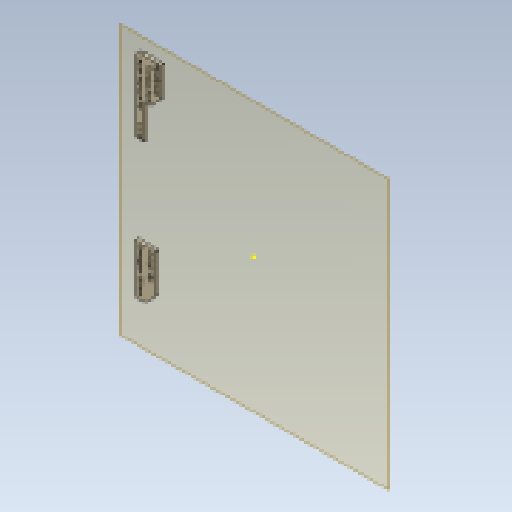
# Autodesk Inventor part: V4-tag
Saved by Autodesk Inventor 2023 (Build 270158030, 158C)
## iProperties
Created: 2024-12-31
Part Number: V4-tag
Material: Generic
Document SubType Name: Modeling
Designer: Imogen Heard
Density: 1 g/cm^3
Appearance: Default
Author: Imogen Heard
Autodesk Inventor part; units mm, degrees
(part 1 of 2)
ref_plane "YZ Plane" through (0, 0, 0) normal (1, 0, 0) x (0, 1, 0)
ref_plane "XZ Plane" through (0, 0, 0) normal (0, 1, 0) x (-1, 0, 0)
ref_plane "XY Plane" through (0, 0, 0) normal (0, 0, 1) x (1, 0, 0)
ref_plane "Work Plane1" through (0, 0, 0) normal (0, 0, 1) x (1, 0, 0)
sketch "Sketch1" plane through (0, 0, 0) normal (0, 0, 1) x (1, 0, 0)
  arc A0 (-110, 115) -> (-115, 110) centre (-110, 110) ccw projected
  line L0 (-115, 110) -> (-115, -110) projected
  arc A1 (-115, -110) -> (-110, -115) centre (-110, -110) ccw projected
  line L1 (-110, -115) -> (110, -115) projected
  arc A2 (110, -115) -> (115, -110) centre (110, -110) ccw projected
  line L2 (115, -110) -> (115, 110) projected
  arc A3 (115, 110) -> (110, 115) centre (110, 110) ccw projected
  line L3 (110, 115) -> (-110, 115) projected
  line L4 (-112, -107) -> (-112, 107) projected
  arc A4 (-107, 112) -> (-112, 107) centre (-107, 107) ccw projected
  line L5 (-107, 112) -> (107, 112) projected
  arc A5 (112, 107) -> (107, 112) centre (107, 107) ccw projected
  line L6 (112, 107) -> (112, -107) projected
  arc A6 (107, -112) -> (112, -107) centre (107, -107) ccw projected
  line L7 (107, -112) -> (-107, -112) projected
  arc A7 (-112, -107) -> (-107, -112) centre (-107, -107) ccw projected
  line L8 (-112, 106.9171) -> (-103.6459, 106.9171)
  line L9 (-103.6459, 106.9171) -> (-103.6459, 42)
  line L10 (-103.6459, 42) -> (-112, 42)
  line L11 (-112, 42) -> (-112, 106.9171)
  line L12 (-87.4562, 112) -> (-103.6459, 112)
  line L13 (-103.6459, 112) -> (-103.6459, 74.4586)
  line L14 (-103.6459, 74.4586) -> (-87.4562, 74.4586)
  line L15 (-87.4562, 74.4586) -> (-87.4562, 112)
  line L16 (-112, -88.3406) -> (-103.6459, -88.3406)
  line L17 (-103.6459, -88.3406) -> (-103.6459, -20.4572)
  line L18 (-103.6459, -20.4572) -> (-112, -20.4572)
  line L19 (-112, -20.4572) -> (-112, -88.3406)
  line L20 (-103.6459, -88.3406) -> (-92.5687, -88.3406)
  line L21 (-92.5687, -88.3406) -> (-92.5687, -42.0436)
  line L22 (-92.5687, -42.0436) -> (-103.6459, -42.0436)
  line L23 (-103.6459, -42.0436) -> (-103.6459, -88.3406)
  line L24 (-103.6459, -42.0436) -> (-112, -42.0436)
  point P0 (0, 0)
  point P1 (-112, 42)
  dimension "d0" = 19.4313
  dimension "d1" = 23.6594
  dimension "d2" = 67.8835
  dimension "d3" = 8.3541
  dimension "d4" = 46.2971
  dimension "d5" = 37.5414
  dimension "d6" = 24.5438
  dimension "d7" = 70
  constraints: 34 end point, 8 parallel, 5 perpendicular, 4 horizontal, 3 point on line, 1 midpoint, 1 vertical alignment
  measures "d0" distance between parallel lines of L4 L21
  measures "d1" distance between parallel lines of L7 L20
  measures "d2" distance between parallel lines of L16 L18
  measures "d3" distance between parallel lines of L4 L17
  measures "d4" distance between parallel lines of L20 L22
  measures "d5" distance between parallel lines of L14 L5
  measures "d6" distance between parallel lines of L4 L15
  measures "d7" distance between parallel lines of L5 L10
ref_plane "Work Plane2" through (-115, -115, -3) normal (0, 0, -1) x (0, 1, 0)
extrude "Extrusion1" add sketch "Sketch1" against normal up to surface (3 mm away) contours L4 L24 L17 L16 | L17 L22 L21 L20 | L4 L8 L9 L10 | L4 A4 L5 L13 L8 | L13 L5 L15 L14 L9
sketch "Sketch2" plane through (0, 0, 0) normal (0, 0, 1) x (1, 0, 0)
  line L0 (-96.6325, 106.512) -> (-96.6325, 80.11) construction
  line L1 (-96.6325, 80.11) -> (-101.6576, 80.11) construction
  line L2 (-101.6576, 80.11) -> (-101.6576, 106.512) construction
  line L3 (-101.6576, 106.512) -> (-96.6325, 106.512) construction
  line L4 (-104.2392, -43.9733) -> (-104.2392, -87.8328) construction
  line L5 (-104.2392, -87.8328) -> (-109.5674, -87.8328) construction
  line L6 (-109.5674, -87.8328) -> (-109.5674, -43.9733) construction
  line L7 (-109.5674, -43.9733) -> (-104.2392, -43.9733) construction
  line L8 (-105.1294, 107.7909) -> (-105.1294, 58.4425) construction
  line L9 (-105.1294, 58.4425) -> (-111.7495, 58.4425) construction
  line L10 (-111.7495, 58.4425) -> (-111.7495, 107.7909) construction
  line L11 (-111.7495, 107.7909) -> (-105.1294, 107.7909) construction
  line L12 (-111.4099, 55.2755) -> (-105.5419, 55.2755) construction
  line L13 (-105.5419, 55.2755) -> (-105.5419, 39.3946) construction
  line L14 (-105.5419, 39.3946) -> (-111.4099, 39.3946) construction
  line L15 (-111.4099, 39.3946) -> (-111.4099, 55.2755) construction
  line L16 (-88.9713, 111.3431) -> (-88.9713, 84.8277) construction
  line L17 (-88.9713, 84.8277) -> (-94.2996, 84.8277) construction
  line L18 (-94.2996, 84.8277) -> (-94.2996, 111.3431) construction
  line L19 (-94.2996, 111.3431) -> (-88.9713, 111.3431) construction
  line L20 (-101.2537, -44.3446) -> (-95.3445, -44.3446) construction
  line L21 (-95.3445, -44.3446) -> (-95.3445, -74.0743) construction
  line L22 (-95.3445, -74.0743) -> (-101.2537, -74.0743) construction
  line L23 (-101.2537, -74.0743) -> (-101.2537, -44.3446) construction
  line L24 (-94.1942, 106.5497) -> (-94.1942, 107.2142)
  line L25 (-94.1942, 107.2142) -> (-89.8871, 107.2142)
  line L26 (-89.8871, 107.2142) -> (-92.8166, 108.5189)
  line L27 (-92.8166, 108.5189) -> (-92.8166, 108.9241)
  line L28 (-92.8166, 108.9241) -> (-89.8871, 110.2166)
  line L29 (-89.8871, 110.2166) -> (-94.1942, 110.2166)
  line L30 (-94.1942, 110.2166) -> (-94.1942, 110.8366)
  line L31 (-94.1942, 110.8366) -> (-89.1942, 110.8366)
  line L32 (-89.1942, 110.8366) -> (-89.1942, 109.929)
  line L33 (-89.1942, 109.929) -> (-91.9778, 108.681)
  line L34 (-91.9778, 108.681) -> (-89.1942, 107.4735)
  line L35 (-89.1942, 107.4735) -> (-89.1942, 106.5497)
  line L36 (-89.1942, 106.5497) -> (-94.1942, 106.5497)
  spline S0 degree 2 poles (-94.2793, 103.9565) (-94.2793, 104.856) (-93.2704, 105.8447) (-92.3384, 105.8447) knots 0 0 0 1 2 2 2
  spline S1 degree 2 poles (-92.3384, 105.8447) (-91.4227, 105.8447) (-90.3368, 104.8844) (-90.3368, 104.1105) knots 0 0 0 1 2 2 2
  spline S2 degree 2 poles (-90.3368, 104.1105) (-90.3368, 103.762) (-90.5394, 103.2231) (-90.7542, 103.0246) knots 0 0 0 1 2 2 2
  spline S3 degree 2 poles (-90.7542, 103.0246) (-90.9689, 102.822) (-91.5889, 102.6072) (-92.0386, 102.6072) knots 0 0 0 1 2 2 2
  line L37 (-92.0386, 102.6072) -> (-92.383, 102.6072)
  line L38 (-92.383, 102.6072) -> (-92.383, 105.2045)
  spline S4 degree 2 poles (-92.383, 105.2045) (-93.0354, 105.2045) (-93.7282, 104.5481) (-93.7282, 103.9646) knots 0 0 0 1 2 2 2
  spline S5 degree 2 poles (-93.7282, 103.9646) (-93.7282, 103.758) (-93.635, 103.3568) (-93.5621, 103.1948) knots 0 0 0 1 2 2 2
  spline S6 degree 2 poles (-93.5621, 103.1948) (-93.4811, 103.0246) (-93.3393, 102.7896) (-93.2744, 102.7126) knots 0 0 0 1 2 2 2
  line L39 (-93.2744, 102.7126) -> (-93.2744, 102.6761)
  line L40 (-93.2744, 102.6761) -> (-93.9632, 102.6761)
  spline S7 degree 2 poles (-93.9632, 102.6761) (-94.0078, 102.7855) (-94.1375, 103.1178) (-94.1739, 103.2474) knots 0 0 0 1 2 2 2
  spline S8 degree 2 poles (-94.1739, 103.2474) (-94.2266, 103.4298) (-94.2793, 103.7296) (-94.2793, 103.9565) knots 0 0 0 1 2 2 2
  spline S9 degree 2 poles (-91.9008, 103.2231) (-91.6456, 103.2312) (-91.2728, 103.3366) (-91.1472, 103.4379) knots 0 0 0 1 2 2 2
  spline S10 degree 2 poles (-91.1472, 103.4379) (-91.0054, 103.5473) (-90.8555, 103.8917) (-90.8555, 104.147) knots 0 0 0 1 2 2 2
  spline S11 degree 2 poles (-90.8555, 104.147) (-90.8555, 104.3982) (-91.0054, 104.7507) (-91.1513, 104.8965) knots 0 0 0 1 2 2 2
  spline S12 degree 2 poles (-91.1513, 104.8965) (-91.3012, 105.0384) (-91.6618, 105.1842) (-91.9008, 105.2045) knots 0 0 0 1 2 2 2
  line L41 (-91.9008, 105.2045) -> (-91.9008, 103.2231)
  line L42 (-94.1942, 99.0821) -> (-94.1942, 99.7142)
  line L43 (-94.1942, 99.7142) -> (-93.8133, 99.7142)
  spline S13 degree 2 poles (-93.8133, 99.7142) (-93.9349, 99.8601) (-94.097, 100.0748) (-94.1658, 100.2207) knots 0 0 0 1 2 2 2
  spline S14 degree 2 poles (-94.1658, 100.2207) (-94.2307, 100.3544) (-94.2996, 100.6421) (-94.2996, 100.8325) knots 0 0 0 1 2 2 2
  spline S15 degree 2 poles (-94.2996, 100.8325) (-94.2996, 101.1405) (-94.0443, 101.6591) (-93.7971, 101.8414) knots 0 0 0 1 2 2 2
  spline S16 degree 2 poles (-93.7971, 101.8414) (-93.55, 102.0238) (-92.8206, 102.2264) (-92.3466, 102.2264) knots 0 0 0 1 2 2 2
  spline S17 degree 2 poles (-92.3466, 102.2264) (-91.8522, 102.2264) (-91.131, 101.9711) (-90.8595, 101.7483) knots 0 0 0 1 2 2 2
  spline S18 degree 2 poles (-90.8595, 101.7483) (-90.6164, 101.5416) (-90.3368, 100.9622) (-90.3368, 100.6421) knots 0 0 0 1 2 2 2
  spline S19 degree 2 poles (-90.3368, 100.6421) (-90.3368, 100.3625) (-90.4624, 99.9452) (-90.5921, 99.7142) knots 0 0 0 1 2 2 2
  line L44 (-90.5921, 99.7142) -> (-88.9713, 99.7142)
  line L45 (-88.9713, 99.7142) -> (-88.9713, 99.0821)
  line L46 (-88.9713, 99.0821) -> (-94.1942, 99.0821)
  line L47 (-93.2825, 99.7142) -> (-91.1148, 99.7142)
  spline S20 degree 2 poles (-91.1148, 99.7142) (-91.0013, 99.9492) (-90.9162, 100.322) (-90.9162, 100.5367) knots 0 0 0 1 2 2 2
  spline S21 degree 2 poles (-90.9162, 100.5367) (-90.9162, 101.023) (-91.6456, 101.574) (-92.3344, 101.574) knots 0 0 0 1 2 2 2
  spline S22 degree 2 poles (-92.3344, 101.574) (-92.9989, 101.574) (-93.6999, 101.1526) (-93.6999, 100.6867) knots 0 0 0 1 2 2 2
  spline S23 degree 2 poles (-93.6999, 100.6867) (-93.6999, 100.4395) (-93.473, 99.9371) (-93.2825, 99.7142) knots 0 0 0 1 2 2 2
  line L48 (-94.1942, 97.5222) -> (-94.1942, 98.1542)
  line L49 (-94.1942, 98.1542) -> (-90.4422, 98.1542)
  line L50 (-90.4422, 98.1542) -> (-90.4422, 97.5222)
  line L51 (-90.4422, 97.5222) -> (-94.1942, 97.5222)
  line L52 (-89.8182, 97.4776) -> (-89.8182, 98.1948)
  line L53 (-89.8182, 98.1948) -> (-89.1618, 98.1948)
  line L54 (-89.1618, 98.1948) -> (-89.1618, 97.4776)
  line L55 (-89.1618, 97.4776) -> (-89.8182, 97.4776)
  spline S24 degree 2 poles (-94.2793, 94.9654) (-94.2793, 95.8649) (-93.2704, 96.8536) (-92.3384, 96.8536) knots 0 0 0 1 2 2 2
  spline S25 degree 2 poles (-92.3384, 96.8536) (-91.4227, 96.8536) (-90.3368, 95.8933) (-90.3368, 95.1194) knots 0 0 0 1 2 2 2
  spline S26 degree 2 poles (-90.3368, 95.1194) (-90.3368, 94.7709) (-90.5394, 94.232) (-90.7542, 94.0335) knots 0 0 0 1 2 2 2
  spline S27 degree 2 poles (-90.7542, 94.0335) (-90.9689, 93.8309) (-91.5889, 93.6162) (-92.0386, 93.6162) knots 0 0 0 1 2 2 2
  line L56 (-92.0386, 93.6162) -> (-92.383, 93.6162)
  line L57 (-92.383, 93.6162) -> (-92.383, 96.2134)
  spline S28 degree 2 poles (-92.383, 96.2134) (-93.0354, 96.2134) (-93.7282, 95.557) (-93.7282, 94.9735) knots 0 0 0 1 2 2 2
  spline S29 degree 2 poles (-93.7282, 94.9735) (-93.7282, 94.7669) (-93.635, 94.3658) (-93.5621, 94.2037) knots 0 0 0 1 2 2 2
  spline S30 degree 2 poles (-93.5621, 94.2037) (-93.4811, 94.0335) (-93.3393, 93.7985) (-93.2744, 93.7215) knots 0 0 0 1 2 2 2
  line L58 (-93.2744, 93.7215) -> (-93.2744, 93.685)
  line L59 (-93.2744, 93.685) -> (-93.9632, 93.685)
  spline S31 degree 2 poles (-93.9632, 93.685) (-94.0078, 93.7944) (-94.1375, 94.1267) (-94.1739, 94.2564) knots 0 0 0 1 2 2 2
  spline S32 degree 2 poles (-94.1739, 94.2564) (-94.2266, 94.4387) (-94.2793, 94.7385) (-94.2793, 94.9654) knots 0 0 0 1 2 2 2
  spline S33 degree 2 poles (-91.9008, 94.232) (-91.6456, 94.2401) (-91.2728, 94.3455) (-91.1472, 94.4468) knots 0 0 0 1 2 2 2
  spline S34 degree 2 poles (-91.1472, 94.4468) (-91.0054, 94.5562) (-90.8555, 94.9006) (-90.8555, 95.1559) knots 0 0 0 1 2 2 2
  spline S35 degree 2 poles (-90.8555, 95.1559) (-90.8555, 95.4071) (-91.0054, 95.7596) (-91.1513, 95.9055) knots 0 0 0 1 2 2 2
  spline S36 degree 2 poles (-91.1513, 95.9055) (-91.3012, 96.0473) (-91.6618, 96.1931) (-91.9008, 96.2134) knots 0 0 0 1 2 2 2
  line L60 (-91.9008, 96.2134) -> (-91.9008, 94.232)
  line L61 (-90.4422, 90.0303) -> (-94.1942, 91.4444)
  line L62 (-94.1942, 91.4444) -> (-94.1942, 92.0116)
  line L63 (-94.1942, 92.0116) -> (-90.4422, 93.4136)
  line L64 (-90.4422, 93.4136) -> (-90.4422, 92.7288)
  line L65 (-90.4422, 92.7288) -> (-93.3312, 91.7037)
  line L66 (-93.3312, 91.7037) -> (-90.4422, 90.6867)
  line L67 (-90.4422, 90.6867) -> (-90.4422, 90.0303)
  spline S37 degree 2 poles (-93.7971, 87.4614) (-93.8538, 87.5384) (-94.0564, 87.7977) (-94.1172, 87.9192) knots 0 0 0 1 2 2 2
  spline S38 degree 2 poles (-94.1172, 87.9192) (-94.2064, 88.0854) (-94.2996, 88.3974) (-94.2996, 88.681) knots 0 0 0 1 2 2 2
  spline S39 degree 2 poles (-94.2996, 88.681) (-94.2996, 88.9119) (-94.1253, 89.3293) (-93.9673, 89.4873) knots 0 0 0 1 2 2 2
  spline S40 degree 2 poles (-93.9673, 89.4873) (-93.8133, 89.6372) (-93.3595, 89.8196) (-93.1083, 89.8196) knots 0 0 0 1 2 2 2
  spline S41 degree 2 poles (-93.1083, 89.8196) (-92.7193, 89.8196) (-92.1683, 89.4914) (-92.0102, 89.1348) knots 0 0 0 1 2 2 2
  spline S42 degree 2 poles (-92.0102, 89.1348) (-91.8644, 88.8188) (-91.755, 87.9598) (-91.7266, 87.4614) knots 0 0 0 1 2 2 2
  line L68 (-91.7266, 87.4614) -> (-91.6051, 87.4614)
  spline S43 degree 2 poles (-91.6051, 87.4614) (-91.3863, 87.4614) (-91.1148, 87.5951) (-91.0378, 87.7166) knots 0 0 0 1 2 2 2
  spline S44 degree 2 poles (-91.0378, 87.7166) (-90.9608, 87.8382) (-90.9122, 88.1867) (-90.9122, 88.373) knots 0 0 0 1 2 2 2
  spline S45 degree 2 poles (-90.9122, 88.373) (-90.9122, 88.5918) (-91.0419, 89.1834) (-91.1675, 89.4792) knots 0 0 0 1 2 2 2
  line L69 (-91.1675, 89.4792) -> (-91.1675, 89.5157)
  line L70 (-91.1675, 89.5157) -> (-90.5232, 89.5157)
  spline S46 degree 2 poles (-90.5232, 89.5157) (-90.4746, 89.3414) (-90.353, 88.6891) (-90.353, 88.369) knots 0 0 0 1 2 2 2
  spline S47 degree 2 poles (-90.353, 88.369) (-90.353, 87.98) (-90.4746, 87.4492) (-90.6326, 87.2385) knots 0 0 0 1 2 2 2
  spline S48 degree 2 poles (-90.6326, 87.2385) (-90.7866, 87.0319) (-91.2769, 86.8293) (-91.6294, 86.8293) knots 0 0 0 1 2 2 2
  line L71 (-91.6294, 86.8293) -> (-94.1942, 86.8293)
  line L72 (-94.1942, 86.8293) -> (-94.1942, 87.4614)
  line L73 (-94.1942, 87.4614) -> (-93.7971, 87.4614)
  line L74 (-93.2704, 87.4614) -> (-92.229, 87.4614)
  spline S49 degree 2 poles (-92.229, 87.4614) (-92.2493, 87.6883) (-92.3182, 88.373) (-92.383, 88.5878) knots 0 0 0 1 2 2 2
  spline S50 degree 2 poles (-92.383, 88.5878) (-92.46, 88.839) (-92.7801, 89.1672) (-93.0637, 89.1672) knots 0 0 0 1 2 2 2
  spline S51 degree 2 poles (-93.0637, 89.1672) (-93.3879, 89.1672) (-93.7161, 88.8025) (-93.7161, 88.4541) knots 0 0 0 1 2 2 2
  spline S52 degree 2 poles (-93.7161, 88.4541) (-93.7161, 88.1583) (-93.4608, 87.6721) (-93.2704, 87.4614) knots 0 0 0 1 2 2 2
  line L75 (-94.1942, 85.2977) -> (-94.1942, 85.9298)
  line L76 (-94.1942, 85.9298) -> (-88.9713, 85.9298)
  line L77 (-88.9713, 85.9298) -> (-88.9713, 85.2977)
  line L78 (-88.9713, 85.2977) -> (-94.1942, 85.2977)
  line L79 (-101.8554, 104.8386) -> (-97.447, 104.8386)
  line L80 (-97.447, 104.8386) -> (-97.447, 106.5161)
  line L81 (-97.447, 106.5161) -> (-96.8554, 106.5161)
  line L82 (-96.8554, 106.5161) -> (-96.8554, 102.4966)
  line L83 (-96.8554, 102.4966) -> (-97.447, 102.4966)
  line L84 (-97.447, 102.4966) -> (-97.447, 104.1741)
  line L85 (-97.447, 104.1741) -> (-101.8554, 104.1741)
  line L86 (-101.8554, 104.1741) -> (-101.8554, 104.8386)
  line L87 (-98.78, 100.0493) -> (-98.78, 100.0817)
  spline S53 degree 2 poles (-98.78, 100.0817) (-98.7598, 100.1547) (-98.7517, 100.3127) (-98.7517, 100.4221) knots 0 0 0 1 2 2 2
  spline S54 degree 2 poles (-98.7517, 100.4221) (-98.7517, 100.6773) (-98.9745, 101.1798) (-99.1933, 101.4067) knots 0 0 0 1 2 2 2
  line L88 (-99.1933, 101.4067) -> (-101.8554, 101.4067)
  line L89 (-101.8554, 101.4067) -> (-101.8554, 102.0388)
  line L90 (-101.8554, 102.0388) -> (-98.1034, 102.0388)
  line L91 (-98.1034, 102.0388) -> (-98.1034, 101.4067)
  line L92 (-98.1034, 101.4067) -> (-98.6625, 101.4067)
  spline S55 degree 2 poles (-98.6625, 101.4067) (-98.3546, 101.0623) (-98.1034, 100.5477) (-98.1034, 100.3046) knots 0 0 0 1 2 2 2
  spline S56 degree 2 poles (-98.1034, 100.3046) (-98.1034, 100.2073) (-98.1115, 100.1101) (-98.1236, 100.0493) knots 0 0 0 1 2 2 2
  line L93 (-98.1236, 100.0493) -> (-98.78, 100.0493)
  spline S57 degree 2 poles (-101.9405, 97.9302) (-101.9405, 98.8297) (-100.9316, 99.8184) (-99.9996, 99.8184) knots 0 0 0 1 2 2 2
  spline S58 degree 2 poles (-99.9996, 99.8184) (-99.0839, 99.8184) (-97.998, 98.8581) (-97.998, 98.0842) knots 0 0 0 1 2 2 2
  spline S59 degree 2 poles (-97.998, 98.0842) (-97.998, 97.7357) (-98.2006, 97.1968) (-98.4154, 96.9983) knots 0 0 0 1 2 2 2
  spline S60 degree 2 poles (-98.4154, 96.9983) (-98.6301, 96.7957) (-99.25, 96.5809) (-99.6998, 96.5809) knots 0 0 0 1 2 2 2
  line L94 (-99.6998, 96.5809) -> (-100.0442, 96.5809)
  line L95 (-100.0442, 96.5809) -> (-100.0442, 99.1782)
  spline S61 degree 2 poles (-100.0442, 99.1782) (-100.6966, 99.1782) (-101.3894, 98.5218) (-101.3894, 97.9383) knots 0 0 0 1 2 2 2
  spline S62 degree 2 poles (-101.3894, 97.9383) (-101.3894, 97.7316) (-101.2962, 97.3305) (-101.2233, 97.1684) knots 0 0 0 1 2 2 2
  spline S63 degree 2 poles (-101.2233, 97.1684) (-101.1423, 96.9983) (-101.0005, 96.7632) (-100.9356, 96.6863) knots 0 0 0 1 2 2 2
  line L96 (-100.9356, 96.6863) -> (-100.9356, 96.6498)
  line L97 (-100.9356, 96.6498) -> (-101.6244, 96.6498)
  spline S64 degree 2 poles (-101.6244, 96.6498) (-101.669, 96.7592) (-101.7987, 97.0914) (-101.8351, 97.2211) knots 0 0 0 1 2 2 2
  spline S65 degree 2 poles (-101.8351, 97.2211) (-101.8878, 97.4034) (-101.9405, 97.7033) (-101.9405, 97.9302) knots 0 0 0 1 2 2 2
  spline S66 degree 2 poles (-99.562, 97.1968) (-99.3068, 97.2049) (-98.934, 97.3102) (-98.8084, 97.4115) knots 0 0 0 1 2 2 2
  spline S67 degree 2 poles (-98.8084, 97.4115) (-98.6666, 97.5209) (-98.5167, 97.8654) (-98.5167, 98.1206) knots 0 0 0 1 2 2 2
  spline S68 degree 2 poles (-98.5167, 98.1206) (-98.5167, 98.3718) (-98.6666, 98.7244) (-98.8124, 98.8702) knots 0 0 0 1 2 2 2
  spline S69 degree 2 poles (-98.8124, 98.8702) (-98.9624, 99.012) (-99.323, 99.1579) (-99.562, 99.1782) knots 0 0 0 1 2 2 2
  line L98 (-99.562, 99.1782) -> (-99.562, 97.1968)
  spline S70 degree 2 poles (-99.9186, 92.7965) (-100.8384, 92.7965) (-101.9607, 93.6879) (-101.9607, 94.3605) knots 0 0 0 1 2 2 2
  spline S71 degree 2 poles (-101.9607, 94.3605) (-101.9607, 94.6644) (-101.8108, 95.0979) (-101.6812, 95.3086) knots 0 0 0 1 2 2 2
  line L99 (-101.6812, 95.3086) -> (-101.8554, 95.3491)
  line L100 (-101.8554, 95.3491) -> (-101.8554, 95.9407)
  line L101 (-101.8554, 95.9407) -> (-96.6325, 95.9407)
  line L102 (-96.6325, 95.9407) -> (-96.6325, 95.3086)
  line L103 (-96.6325, 95.3086) -> (-98.4964, 95.3086)
  spline S72 degree 2 poles (-98.4964, 95.3086) (-98.2816, 95.0696) (-97.998, 94.5145) (-97.998, 94.162) knots 0 0 0 1 2 2 2
  spline S73 degree 2 poles (-97.998, 94.162) (-97.998, 93.5258) (-99.015, 92.7965) (-99.9186, 92.7965) knots 0 0 0 1 2 2 2
  spline S74 degree 2 poles (-99.9672, 93.4488) (-99.2946, 93.4488) (-98.5977, 93.8581) (-98.5977, 94.3119) knots 0 0 0 1 2 2 2
  spline S75 degree 2 poles (-98.5977, 94.3119) (-98.5977, 94.5671) (-98.8408, 95.0939) (-99.0272, 95.3086) knots 0 0 0 1 2 2 2
  line L104 (-99.0272, 95.3086) -> (-101.1787, 95.3086)
  spline S76 degree 2 poles (-101.1787, 95.3086) (-101.2962, 95.0696) (-101.3935, 94.7008) (-101.3935, 94.482) knots 0 0 0 1 2 2 2
  spline S77 degree 2 poles (-101.3935, 94.482) (-101.3935, 93.9999) (-100.7087, 93.4488) (-99.9672, 93.4488) knots 0 0 0 1 2 2 2
  line L105 (-101.8554, 89.2227) -> (-101.8554, 89.8548)
  line L106 (-101.8554, 89.8548) -> (-101.4421, 89.8548)
  spline S78 degree 2 poles (-101.4421, 89.8548) (-101.6974, 90.1466) (-101.9607, 90.6692) (-101.9607, 90.9934) knots 0 0 0 1 2 2 2
  spline S79 degree 2 poles (-101.9607, 90.9934) (-101.9607, 91.2365) (-101.7987, 91.6701) (-101.6244, 91.8281) knots 0 0 0 1 2 2 2
  spline S80 degree 2 poles (-101.6244, 91.8281) (-101.4502, 91.9902) (-100.9194, 92.1684) (-100.5385, 92.1684) knots 0 0 0 1 2 2 2
  line L107 (-100.5385, 92.1684) -> (-98.1034, 92.1684)
  line L108 (-98.1034, 92.1684) -> (-98.1034, 91.5363)
  line L109 (-98.1034, 91.5363) -> (-100.2428, 91.5363)
  spline S81 degree 2 poles (-100.2428, 91.5363) (-100.5426, 91.5363) (-100.9356, 91.4918) (-101.0815, 91.4148) knots 0 0 0 1 2 2 2
  spline S82 degree 2 poles (-101.0815, 91.4148) (-101.2274, 91.3378) (-101.3611, 91.0744) (-101.3611, 90.8273) knots 0 0 0 1 2 2 2
  spline S83 degree 2 poles (-101.3611, 90.8273) (-101.3611, 90.5963) (-101.0977, 90.0736) (-100.9073, 89.8548) knots 0 0 0 1 2 2 2
  line L110 (-100.9073, 89.8548) -> (-98.1034, 89.8548)
  line L111 (-98.1034, 89.8548) -> (-98.1034, 89.2227)
  line L112 (-98.1034, 89.2227) -> (-101.8554, 89.2227)
  spline S84 degree 2 poles (-101.9405, 86.8159) (-101.9405, 87.2049) (-101.7014, 87.8491) (-101.4583, 88.0801) knots 0 0 0 1 2 2 2
  spline S85 degree 2 poles (-101.4583, 88.0801) (-101.2193, 88.3111) (-100.4818, 88.5663) (-99.9875, 88.5663) knots 0 0 0 1 2 2 2
  spline S86 degree 2 poles (-99.9875, 88.5663) (-99.4932, 88.5663) (-98.7719, 88.303) (-98.5288, 88.0801) knots 0 0 0 1 2 2 2
  spline S87 degree 2 poles (-98.5288, 88.0801) (-98.2816, 87.8573) (-98.0183, 87.1968) (-98.0183, 86.8159) knots 0 0 0 1 2 2 2
  spline S88 degree 2 poles (-98.0183, 86.8159) (-98.0183, 86.508) (-98.1925, 85.9326) (-98.306, 85.7098) knots 0 0 0 1 2 2 2
  line L113 (-98.306, 85.7098) -> (-99.015, 85.7098)
  line L114 (-99.015, 85.7098) -> (-99.015, 85.7462)
  spline S89 degree 2 poles (-99.015, 85.7462) (-98.9583, 85.8151) (-98.8124, 86.0258) (-98.7355, 86.1757) knots 0 0 0 1 2 2 2
  spline S90 degree 2 poles (-98.7355, 86.1757) (-98.6706, 86.3094) (-98.5693, 86.666) (-98.5693, 86.8281) knots 0 0 0 1 2 2 2
  spline S91 degree 2 poles (-98.5693, 86.8281) (-98.5693, 87.3184) (-99.3108, 87.914) (-99.9875, 87.914) knots 0 0 0 1 2 2 2
  spline S92 degree 2 poles (-99.9875, 87.914) (-100.6479, 87.914) (-101.3894, 87.3386) (-101.3894, 86.8281) knots 0 0 0 1 2 2 2
  spline S93 degree 2 poles (-101.3894, 86.8281) (-101.3894, 86.5201) (-101.1342, 85.961) (-100.9356, 85.7462) knots 0 0 0 1 2 2 2
  line L115 (-100.9356, 85.7462) -> (-100.9356, 85.7098)
  line L116 (-100.9356, 85.7098) -> (-101.6447, 85.7098)
  spline S94 degree 2 poles (-101.6447, 85.7098) (-101.6893, 85.803) (-101.8149, 86.0866) (-101.8432, 86.2) knots 0 0 0 1 2 2 2
  spline S95 degree 2 poles (-101.8432, 86.2) (-101.8919, 86.3621) (-101.9405, 86.6174) (-101.9405, 86.8159) knots 0 0 0 1 2 2 2
  line L117 (-101.8554, 82.1887) -> (-101.8554, 82.8208)
  line L118 (-101.8554, 82.8208) -> (-99.716, 82.8208)
  spline S96 degree 2 poles (-99.716, 82.8208) (-99.4567, 82.8208) (-99.011, 82.8694) (-98.8773, 82.9423) knots 0 0 0 1 2 2 2
  spline S97 degree 2 poles (-98.8773, 82.9423) (-98.7355, 83.0193) (-98.5977, 83.2949) (-98.5977, 83.5299) knots 0 0 0 1 2 2 2
  spline S98 degree 2 poles (-98.5977, 83.5299) (-98.5977, 83.7649) (-98.8489, 84.2632) (-99.0515, 84.5023) knots 0 0 0 1 2 2 2
  line L119 (-99.0515, 84.5023) -> (-101.8554, 84.5023)
  line L120 (-101.8554, 84.5023) -> (-101.8554, 85.1344)
  line L121 (-101.8554, 85.1344) -> (-96.6325, 85.1344)
  line L122 (-96.6325, 85.1344) -> (-96.6325, 84.5023)
  line L123 (-96.6325, 84.5023) -> (-98.5207, 84.5023)
  spline S99 degree 2 poles (-98.5207, 84.5023) (-98.2654, 84.2187) (-97.998, 83.6717) (-97.998, 83.3637) knots 0 0 0 1 2 2 2
  spline S100 degree 2 poles (-97.998, 83.3637) (-97.998, 82.8127) (-98.7274, 82.1887) (-99.4202, 82.1887) knots 0 0 0 1 2 2 2
  line L124 (-99.4202, 82.1887) -> (-101.8554, 82.1887)
  spline S101 degree 2 poles (-101.9405, 79.6725) (-101.9405, 80.572) (-100.9316, 81.5607) (-99.9996, 81.5607) knots 0 0 0 1 2 2 2
  spline S102 degree 2 poles (-99.9996, 81.5607) (-99.0839, 81.5607) (-97.998, 80.6004) (-97.998, 79.8265) knots 0 0 0 1 2 2 2
  spline S103 degree 2 poles (-97.998, 79.8265) (-97.998, 79.478) (-98.2006, 78.9391) (-98.4154, 78.7406) knots 0 0 0 1 2 2 2
  spline S104 degree 2 poles (-98.4154, 78.7406) (-98.6301, 78.538) (-99.25, 78.3232) (-99.6998, 78.3232) knots 0 0 0 1 2 2 2
  line L125 (-99.6998, 78.3232) -> (-100.0442, 78.3232)
  line L126 (-100.0442, 78.3232) -> (-100.0442, 80.9205)
  spline S105 degree 2 poles (-100.0442, 80.9205) (-100.6966, 80.9205) (-101.3894, 80.2641) (-101.3894, 79.6806) knots 0 0 0 1 2 2 2
  spline S106 degree 2 poles (-101.3894, 79.6806) (-101.3894, 79.4739) (-101.2962, 79.0728) (-101.2233, 78.9107) knots 0 0 0 1 2 2 2
  spline S107 degree 2 poles (-101.2233, 78.9107) (-101.1423, 78.7406) (-101.0005, 78.5055) (-100.9356, 78.4286) knots 0 0 0 1 2 2 2
  line L127 (-100.9356, 78.4286) -> (-100.9356, 78.3921)
  line L128 (-100.9356, 78.3921) -> (-101.6244, 78.3921)
  spline S108 degree 2 poles (-101.6244, 78.3921) (-101.669, 78.5015) (-101.7987, 78.8338) (-101.8351, 78.9634) knots 0 0 0 1 2 2 2
  spline S109 degree 2 poles (-101.8351, 78.9634) (-101.8878, 79.1457) (-101.9405, 79.4456) (-101.9405, 79.6725) knots 0 0 0 1 2 2 2
  spline S110 degree 2 poles (-99.562, 78.9391) (-99.3068, 78.9472) (-98.934, 79.0526) (-98.8084, 79.1538) knots 0 0 0 1 2 2 2
  spline S111 degree 2 poles (-98.8084, 79.1538) (-98.6666, 79.2632) (-98.5167, 79.6077) (-98.5167, 79.8629) knots 0 0 0 1 2 2 2
  spline S112 degree 2 poles (-98.5167, 79.8629) (-98.5167, 80.1141) (-98.6666, 80.4667) (-98.8124, 80.6125) knots 0 0 0 1 2 2 2
  spline S113 degree 2 poles (-98.8124, 80.6125) (-98.9624, 80.7543) (-99.323, 80.9002) (-99.562, 80.9205) knots 0 0 0 1 2 2 2
  line L129 (-99.562, 80.9205) -> (-99.562, 78.9391)
  spline S114 degree 2 poles (-101.9283, 76.5485) (-101.9283, 77.0631) (-101.3408, 77.6425) (-100.7047, 77.6425) knots 0 0 0 1 2 2 2
  line L130 (-100.7047, 77.6425) -> (-98.6261, 77.6425)
  line L131 (-98.6261, 77.6425) -> (-98.6261, 78.0679)
  line L132 (-98.6261, 78.0679) -> (-98.1034, 78.0679)
  line L133 (-98.1034, 78.0679) -> (-98.1034, 77.6425)
  line L134 (-98.1034, 77.6425) -> (-97.0256, 77.6425)
  line L135 (-97.0256, 77.6425) -> (-97.0256, 77.0104)
  line L136 (-97.0256, 77.0104) -> (-98.1034, 77.0104)
  line L137 (-98.1034, 77.0104) -> (-98.1034, 75.8475)
  line L138 (-98.1034, 75.8475) -> (-98.6261, 75.8475)
  line L139 (-98.6261, 75.8475) -> (-98.6261, 77.0104)
  line L140 (-98.6261, 77.0104) -> (-100.4129, 77.0104)
  spline S115 degree 2 poles (-100.4129, 77.0104) (-100.6966, 77.0104) (-101.0086, 76.9902) (-101.1423, 76.9213) knots 0 0 0 1 2 2 2
  spline S116 degree 2 poles (-101.1423, 76.9213) (-101.2598, 76.8645) (-101.3773, 76.6093) (-101.3773, 76.3905) knots 0 0 0 1 2 2 2
  spline S117 degree 2 poles (-101.3773, 76.3905) (-101.3773, 76.2365) (-101.2841, 75.9488) (-101.2557, 75.884) knots 0 0 0 1 2 2 2
  line L141 (-101.2557, 75.884) -> (-101.2557, 75.8475)
  line L142 (-101.2557, 75.8475) -> (-101.823, 75.8475)
  spline S118 degree 2 poles (-101.823, 75.8475) (-101.8716, 76.0258) (-101.9283, 76.3905) (-101.9283, 76.5485) knots 0 0 0 1 2 2 2
  spline S119 degree 2 poles (-108.1051, 104.6726) (-108.4033, 104.6726) (-108.8604, 104.8995) (-109.0095, 105.0875) knots 0 0 0 1 2 2 2
  spline S120 degree 2 poles (-109.0095, 105.0875) (-109.1845, 105.3144) (-109.3336, 105.8298) (-109.3336, 106.2383) knots 0 0 0 1 2 2 2
  line L143 (-109.3336, 106.2383) -> (-109.3336, 107.3858)
  line L144 (-109.3336, 107.3858) -> (-105.3336, 107.3858)
  line L145 (-105.3336, 107.3858) -> (-105.3336, 106.3258)
  spline S121 degree 2 poles (-105.3336, 106.3258) (-105.3336, 105.8979) (-105.3887, 105.47) (-105.4957, 105.2755) knots 0 0 0 1 2 2 2
  spline S122 degree 2 poles (-105.4957, 105.2755) (-105.6092, 105.0584) (-105.9819, 104.8606) (-106.2348, 104.8606) knots 0 0 0 1 2 2 2
  spline S123 degree 2 poles (-106.2348, 104.8606) (-106.5168, 104.8606) (-106.9641, 105.1589) (-107.0905, 105.4214) knots 0 0 0 1 2 2 2
  line L146 (-107.0905, 105.4214) -> (-107.11, 105.4214)
  spline S124 degree 2 poles (-107.11, 105.4214) (-107.2072, 105.0649) (-107.7226, 104.6726) (-108.1051, 104.6726) knots 0 0 0 1 2 2 2
  spline S125 degree 2 poles (-108.1278, 105.2269) (-107.9009, 105.2269) (-107.6092, 105.3566) (-107.5054, 105.5511) knots 0 0 0 1 2 2 2
  spline S126 degree 2 poles (-107.5054, 105.5511) (-107.4406, 105.6775) (-107.4017, 105.9757) (-107.4017, 106.2512) knots 0 0 0 1 2 2 2
  line L147 (-107.4017, 106.2512) -> (-107.4017, 106.8542)
  line L148 (-107.4017, 106.8542) -> (-108.8798, 106.8542)
  line L149 (-108.8798, 106.8542) -> (-108.8798, 106.423)
  spline S127 degree 2 poles (-108.8798, 106.423) (-108.8798, 106.073) (-108.815, 105.671) (-108.7113, 105.5154) knots 0 0 0 1 2 2 2
  spline S128 degree 2 poles (-108.7113, 105.5154) (-108.6043, 105.3663) (-108.3385, 105.2269) (-108.1278, 105.2269) knots 0 0 0 1 2 2 2
  spline S129 degree 2 poles (-106.3093, 105.4149) (-106.1667, 105.4149) (-105.9528, 105.5122) (-105.8912, 105.6191) knots 0 0 0 1 2 2 2
  spline S130 degree 2 poles (-105.8912, 105.6191) (-105.8199, 105.7488) (-105.7874, 106.0632) (-105.7874, 106.3452) knots 0 0 0 1 2 2 2
  line L150 (-105.7874, 106.3452) -> (-105.7874, 106.8542)
  line L151 (-105.7874, 106.8542) -> (-106.9576, 106.8542)
  line L152 (-106.9576, 106.8542) -> (-106.9576, 106.2512)
  spline S131 degree 2 poles (-106.9576, 106.2512) (-106.9576, 106.0016) (-106.9058, 105.765) (-106.8247, 105.6386) knots 0 0 0 1 2 2 2
  spline S132 degree 2 poles (-106.8247, 105.6386) (-106.7469, 105.5154) (-106.4973, 105.4149) (-106.3093, 105.4149) knots 0 0 0 1 2 2 2
  line L153 (-109.3336, 101.8493) -> (-109.3336, 102.355)
  line L154 (-109.3336, 102.355) -> (-109.003, 102.355)
  spline S133 degree 2 poles (-109.003, 102.355) (-109.2072, 102.5884) (-109.4179, 103.0065) (-109.4179, 103.2658) knots 0 0 0 1 2 2 2
  spline S134 degree 2 poles (-109.4179, 103.2658) (-109.4179, 103.4603) (-109.2883, 103.8072) (-109.1489, 103.9336) knots 0 0 0 1 2 2 2
  spline S135 degree 2 poles (-109.1489, 103.9336) (-109.0095, 104.0632) (-108.5849, 104.2059) (-108.2802, 104.2059) knots 0 0 0 1 2 2 2
  line L155 (-108.2802, 104.2059) -> (-106.332, 104.2059)
  line L156 (-106.332, 104.2059) -> (-106.332, 103.7002)
  line L157 (-106.332, 103.7002) -> (-108.0435, 103.7002)
  spline S136 degree 2 poles (-108.0435, 103.7002) (-108.2834, 103.7002) (-108.5978, 103.6645) (-108.7145, 103.6029) knots 0 0 0 1 2 2 2
  spline S137 degree 2 poles (-108.7145, 103.6029) (-108.8312, 103.5414) (-108.9382, 103.3307) (-108.9382, 103.1329) knots 0 0 0 1 2 2 2
  spline S138 degree 2 poles (-108.9382, 103.1329) (-108.9382, 102.9482) (-108.7275, 102.53) (-108.5751, 102.355) knots 0 0 0 1 2 2 2
  line L158 (-108.5751, 102.355) -> (-106.332, 102.355)
  line L159 (-106.332, 102.355) -> (-106.332, 101.8493)
  line L160 (-106.332, 101.8493) -> (-109.3336, 101.8493)
  line L161 (-109.3336, 100.6013) -> (-109.3336, 101.107)
  line L162 (-109.3336, 101.107) -> (-106.332, 101.107)
  line L163 (-106.332, 101.107) -> (-106.332, 100.6013)
  line L164 (-106.332, 100.6013) -> (-109.3336, 100.6013)
  line L165 (-105.8328, 100.5657) -> (-105.8328, 101.1394)
  line L166 (-105.8328, 101.1394) -> (-105.3077, 101.1394)
  line L167 (-105.3077, 101.1394) -> (-105.3077, 100.5657)
  line L168 (-105.3077, 100.5657) -> (-105.8328, 100.5657)
  line L169 (-109.3336, 99.3436) -> (-109.3336, 99.8493)
  line L170 (-109.3336, 99.8493) -> (-105.1554, 99.8493)
  line L171 (-105.1554, 99.8493) -> (-105.1554, 99.3436)
  line L172 (-105.1554, 99.3436) -> (-109.3336, 99.3436)
  line L173 (-109.3336, 96.2934) -> (-109.3336, 96.7991)
  line L174 (-109.3336, 96.7991) -> (-109.0289, 96.7991)
  spline S139 degree 2 poles (-109.0289, 96.7991) (-109.1262, 96.9157) (-109.2558, 97.0875) (-109.311, 97.2042) knots 0 0 0 1 2 2 2
  spline S140 degree 2 poles (-109.311, 97.2042) (-109.3628, 97.3112) (-109.4179, 97.5414) (-109.4179, 97.6937) knots 0 0 0 1 2 2 2
  spline S141 degree 2 poles (-109.4179, 97.6937) (-109.4179, 97.9401) (-109.2137, 98.355) (-109.016, 98.5008) knots 0 0 0 1 2 2 2
  spline S142 degree 2 poles (-109.016, 98.5008) (-108.8182, 98.6467) (-108.2348, 98.8088) (-107.8555, 98.8088) knots 0 0 0 1 2 2 2
  spline S143 degree 2 poles (-107.8555, 98.8088) (-107.4601, 98.8088) (-106.8831, 98.6046) (-106.6659, 98.4263) knots 0 0 0 1 2 2 2
  spline S144 degree 2 poles (-106.6659, 98.4263) (-106.4714, 98.261) (-106.2477, 97.7974) (-106.2477, 97.5414) knots 0 0 0 1 2 2 2
  spline S145 degree 2 poles (-106.2477, 97.5414) (-106.2477, 97.3177) (-106.3482, 96.9838) (-106.452, 96.7991) knots 0 0 0 1 2 2 2
  line L175 (-106.452, 96.7991) -> (-105.1554, 96.7991)
  line L176 (-105.1554, 96.7991) -> (-105.1554, 96.2934)
  line L177 (-105.1554, 96.2934) -> (-109.3336, 96.2934)
  line L178 (-108.6043, 96.7991) -> (-106.8701, 96.7991)
  spline S146 degree 2 poles (-106.8701, 96.7991) (-106.7793, 96.9871) (-106.7113, 97.2853) (-106.7113, 97.4571) knots 0 0 0 1 2 2 2
  spline S147 degree 2 poles (-106.7113, 97.4571) (-106.7113, 97.8461) (-107.2947, 98.2869) (-107.8458, 98.2869) knots 0 0 0 1 2 2 2
  spline S148 degree 2 poles (-107.8458, 98.2869) (-108.3774, 98.2869) (-108.9382, 97.9498) (-108.9382, 97.577) knots 0 0 0 1 2 2 2
  spline S149 degree 2 poles (-108.9382, 97.577) (-108.9382, 97.3793) (-108.7567, 96.9773) (-108.6043, 96.7991) knots 0 0 0 1 2 2 2
  line L179 (-105.3336, 91.0033) -> (-107.5638, 92.355)
  line L180 (-107.5638, 92.355) -> (-109.3336, 92.355)
  line L181 (-109.3336, 92.355) -> (-109.3336, 92.8866)
  line L182 (-109.3336, 92.8866) -> (-107.6189, 92.8866)
  line L183 (-107.6189, 92.8866) -> (-105.3336, 94.2383)
  line L184 (-105.3336, 94.2383) -> (-105.3336, 93.6483)
  line L185 (-105.3336, 93.6483) -> (-107.0938, 92.6175)
  line L186 (-107.0938, 92.6175) -> (-105.3336, 91.5673)
  line L187 (-105.3336, 91.5673) -> (-105.3336, 91.0033)
  spline S150 degree 2 poles (-107.8328, 88.2059) (-108.5913, 88.2059) (-109.4179, 88.9352) (-109.4179, 89.5446) knots 0 0 0 1 2 2 2
  spline S151 degree 2 poles (-109.4179, 89.5446) (-109.4179, 90.1702) (-108.5654, 90.8866) (-107.8328, 90.8866) knots 0 0 0 1 2 2 2
  spline S152 degree 2 poles (-107.8328, 90.8866) (-107.0808, 90.8866) (-106.2477, 90.1475) (-106.2477, 89.5446) knots 0 0 0 1 2 2 2
  spline S153 degree 2 poles (-106.2477, 89.5446) (-106.2477, 88.9352) (-107.0776, 88.2059) (-107.8328, 88.2059) knots 0 0 0 1 2 2 2
  spline S154 degree 2 poles (-107.8328, 88.7277) (-107.2494, 88.7277) (-106.6821, 89.1524) (-106.6821, 89.5446) knots 0 0 0 1 2 2 2
  spline S155 degree 2 poles (-106.6821, 89.5446) (-106.6821, 89.9368) (-107.2494, 90.3647) (-107.8328, 90.3647) knots 0 0 0 1 2 2 2
  spline S156 degree 2 poles (-107.8328, 90.3647) (-108.4001, 90.3647) (-108.9836, 89.9368) (-108.9836, 89.5446) knots 0 0 0 1 2 2 2
  spline S157 degree 2 poles (-108.9836, 89.5446) (-108.9836, 89.1556) (-108.4098, 88.7277) (-107.8328, 88.7277) knots 0 0 0 1 2 2 2
  line L188 (-109.3336, 85.3533) -> (-109.3336, 85.859)
  line L189 (-109.3336, 85.859) -> (-109.003, 85.859)
  spline S158 degree 2 poles (-109.003, 85.859) (-109.2072, 86.0924) (-109.4179, 86.5106) (-109.4179, 86.7699) knots 0 0 0 1 2 2 2
  spline S159 degree 2 poles (-109.4179, 86.7699) (-109.4179, 86.9644) (-109.2883, 87.3112) (-109.1489, 87.4376) knots 0 0 0 1 2 2 2
  spline S160 degree 2 poles (-109.1489, 87.4376) (-109.0095, 87.5673) (-108.5849, 87.7099) (-108.2802, 87.7099) knots 0 0 0 1 2 2 2
  line L190 (-108.2802, 87.7099) -> (-106.332, 87.7099)
  line L191 (-106.332, 87.7099) -> (-106.332, 87.2042)
  line L192 (-106.332, 87.2042) -> (-108.0435, 87.2042)
  spline S161 degree 2 poles (-108.0435, 87.2042) (-108.2834, 87.2042) (-108.5978, 87.1686) (-108.7145, 87.107) knots 0 0 0 1 2 2 2
  spline S162 degree 2 poles (-108.7145, 87.107) (-108.8312, 87.0454) (-108.9382, 86.8347) (-108.9382, 86.637) knots 0 0 0 1 2 2 2
  spline S163 degree 2 poles (-108.9382, 86.637) (-108.9382, 86.4522) (-108.7275, 86.0341) (-108.5751, 85.859) knots 0 0 0 1 2 2 2
  line L193 (-108.5751, 85.859) -> (-106.332, 85.859)
  line L194 (-106.332, 85.859) -> (-106.332, 85.3533)
  line L195 (-106.332, 85.3533) -> (-109.3336, 85.3533)
  line L196 (-106.8733, 83.0292) -> (-106.8733, 83.0551)
  spline S164 degree 2 poles (-106.8733, 83.0551) (-106.8571, 83.1135) (-106.8507, 83.2399) (-106.8507, 83.3274) knots 0 0 0 1 2 2 2
  spline S165 degree 2 poles (-106.8507, 83.3274) (-106.8507, 83.5316) (-107.0289, 83.9336) (-107.204, 84.1151) knots 0 0 0 1 2 2 2
  line L197 (-107.204, 84.1151) -> (-109.3336, 84.1151)
  line L198 (-109.3336, 84.1151) -> (-109.3336, 84.6208)
  line L199 (-109.3336, 84.6208) -> (-106.332, 84.6208)
  line L200 (-106.332, 84.6208) -> (-106.332, 84.1151)
  line L201 (-106.332, 84.1151) -> (-106.7793, 84.1151)
  spline S166 degree 2 poles (-106.7793, 84.1151) (-106.533, 83.8396) (-106.332, 83.4279) (-106.332, 83.2334) knots 0 0 0 1 2 2 2
  spline S167 degree 2 poles (-106.332, 83.2334) (-106.332, 83.1556) (-106.3385, 83.0778) (-106.3482, 83.0292) knots 0 0 0 1 2 2 2
  line L202 (-106.3482, 83.0292) -> (-106.8733, 83.0292)
  spline S168 degree 2 poles (-109.405, 81.8266) (-109.405, 82.1281) (-109.2429, 82.6499) (-109.1521, 82.8217) knots 0 0 0 1 2 2 2
  line L203 (-109.1521, 82.8217) -> (-108.5849, 82.8217)
  line L204 (-108.5849, 82.8217) -> (-108.5849, 82.7958)
  spline S169 degree 2 poles (-108.5849, 82.7958) (-108.6367, 82.731) (-108.7599, 82.5559) (-108.828, 82.4101) knots 0 0 0 1 2 2 2
  spline S170 degree 2 poles (-108.828, 82.4101) (-108.8896, 82.2837) (-108.9803, 81.9725) (-108.9803, 81.8072) knots 0 0 0 1 2 2 2
  spline S171 degree 2 poles (-108.9803, 81.8072) (-108.9803, 81.6872) (-108.9252, 81.4117) (-108.8798, 81.3469) knots 0 0 0 1 2 2 2
  spline S172 degree 2 poles (-108.8798, 81.3469) (-108.8182, 81.2529) (-108.6789, 81.1686) (-108.5362, 81.1686) knots 0 0 0 1 2 2 2
  spline S173 degree 2 poles (-108.5362, 81.1686) (-108.358, 81.1686) (-108.1732, 81.3631) (-108.1116, 81.6127) knots 0 0 0 1 2 2 2
  spline S174 degree 2 poles (-108.1116, 81.6127) (-108.0889, 81.7099) (-108.0241, 82.0211) (-107.9884, 82.154) knots 0 0 0 1 2 2 2
  spline S175 degree 2 poles (-107.9884, 82.154) (-107.8879, 82.4976) (-107.473, 82.8088) (-107.178, 82.8088) knots 0 0 0 1 2 2 2
  spline S176 degree 2 poles (-107.178, 82.8088) (-106.7696, 82.8088) (-106.2607, 82.1961) (-106.2607, 81.6905) knots 0 0 0 1 2 2 2
  spline S177 degree 2 poles (-106.2607, 81.6905) (-106.2607, 81.4409) (-106.3839, 80.9352) (-106.4779, 80.7634) knots 0 0 0 1 2 2 2
  line L205 (-106.4779, 80.7634) -> (-107.0192, 80.7634)
  line L206 (-107.0192, 80.7634) -> (-107.0192, 80.7893)
  spline S178 degree 2 poles (-107.0192, 80.7893) (-106.8636, 80.9838) (-106.6853, 81.4571) (-106.6853, 81.7002) knots 0 0 0 1 2 2 2
  spline S179 degree 2 poles (-106.6853, 81.7002) (-106.6853, 81.9498) (-106.896, 82.2934) (-107.1067, 82.2934) knots 0 0 0 1 2 2 2
  spline S180 degree 2 poles (-107.1067, 82.2934) (-107.298, 82.2934) (-107.4827, 82.0892) (-107.5411, 81.8623) knots 0 0 0 1 2 2 2
  spline S181 degree 2 poles (-107.5411, 81.8623) (-107.5703, 81.752) (-107.6286, 81.4733) (-107.6643, 81.3209) knots 0 0 0 1 2 2 2
  spline S182 degree 2 poles (-107.6643, 81.3209) (-107.7486, 80.9903) (-108.1343, 80.6532) (-108.4682, 80.6532) knots 0 0 0 1 2 2 2
  spline S183 degree 2 poles (-108.4682, 80.6532) (-108.6627, 80.6532) (-109.0063, 80.8055) (-109.1327, 80.9546) knots 0 0 0 1 2 2 2
  spline S184 degree 2 poles (-109.1327, 80.9546) (-109.2656, 81.1135) (-109.405, 81.5187) (-109.405, 81.8266) knots 0 0 0 1 2 2 2
  spline S185 degree 2 poles (-109.4017, 78.8801) (-109.4017, 79.5997) (-108.5946, 80.3906) (-107.849, 80.3906) knots 0 0 0 1 2 2 2
  spline S186 degree 2 poles (-107.849, 80.3906) (-107.1165, 80.3906) (-106.2477, 79.6224) (-106.2477, 79.0033) knots 0 0 0 1 2 2 2
  spline S187 degree 2 poles (-106.2477, 79.0033) (-106.2477, 78.7245) (-106.4098, 78.2934) (-106.5816, 78.1345) knots 0 0 0 1 2 2 2
  spline S188 degree 2 poles (-106.5816, 78.1345) (-106.7534, 77.9725) (-107.2494, 77.8007) (-107.6092, 77.8007) knots 0 0 0 1 2 2 2
  line L207 (-107.6092, 77.8007) -> (-107.8847, 77.8007)
  line L208 (-107.8847, 77.8007) -> (-107.8847, 79.8785)
  spline S189 degree 2 poles (-107.8847, 79.8785) (-108.4066, 79.8785) (-108.9609, 79.3533) (-108.9609, 78.8866) knots 0 0 0 1 2 2 2
  spline S190 degree 2 poles (-108.9609, 78.8866) (-108.9609, 78.7213) (-108.8863, 78.4003) (-108.828, 78.2707) knots 0 0 0 1 2 2 2
  spline S191 degree 2 poles (-108.828, 78.2707) (-108.7631, 78.1345) (-108.6497, 77.9465) (-108.5978, 77.8849) knots 0 0 0 1 2 2 2
  line L209 (-108.5978, 77.8849) -> (-108.5978, 77.8558)
  line L210 (-108.5978, 77.8558) -> (-109.1489, 77.8558)
  spline S192 degree 2 poles (-109.1489, 77.8558) (-109.1845, 77.9433) (-109.2883, 78.2091) (-109.3174, 78.3128) knots 0 0 0 1 2 2 2
  spline S193 degree 2 poles (-109.3174, 78.3128) (-109.3596, 78.4587) (-109.4017, 78.6986) (-109.4017, 78.8801) knots 0 0 0 1 2 2 2
  spline S194 degree 2 poles (-107.499, 78.2934) (-107.2947, 78.2999) (-106.9965, 78.3841) (-106.896, 78.4652) knots 0 0 0 1 2 2 2
  spline S195 degree 2 poles (-106.896, 78.4652) (-106.7826, 78.5527) (-106.6627, 78.8282) (-106.6627, 79.0324) knots 0 0 0 1 2 2 2
  spline S196 degree 2 poles (-106.6627, 79.0324) (-106.6627, 79.2334) (-106.7826, 79.5154) (-106.8993, 79.6321) knots 0 0 0 1 2 2 2
  spline S197 degree 2 poles (-106.8993, 79.6321) (-107.0192, 79.7456) (-107.3077, 79.8623) (-107.499, 79.8785) knots 0 0 0 1 2 2 2
  line L211 (-107.499, 79.8785) -> (-107.499, 78.2934)
  line L212 (-109.3336, 76.7731) -> (-109.3336, 77.2788)
  line L213 (-109.3336, 77.2788) -> (-105.1554, 77.2788)
  line L214 (-105.1554, 77.2788) -> (-105.1554, 76.7731)
  line L215 (-105.1554, 76.7731) -> (-109.3336, 76.7731)
  line L216 (-105.6416, 74.4522) -> (-105.6416, 74.4781)
  spline S198 degree 2 poles (-105.6416, 74.4781) (-105.6157, 74.5462) (-105.5703, 74.7991) (-105.5703, 74.8995) knots 0 0 0 1 2 2 2
  spline S199 degree 2 poles (-105.5703, 74.8995) (-105.5703, 75.2172) (-105.8555, 75.4895) (-106.2315, 75.4895) knots 0 0 0 1 2 2 2
  line L217 (-106.2315, 75.4895) -> (-106.332, 75.4895)
  line L218 (-106.332, 75.4895) -> (-106.332, 74.6532)
  line L219 (-106.332, 74.6532) -> (-106.7502, 74.6532)
  line L220 (-106.7502, 74.6532) -> (-106.7502, 75.4733)
  line L221 (-106.7502, 75.4733) -> (-109.3336, 75.4733)
  line L222 (-109.3336, 75.4733) -> (-109.3336, 75.979)
  line L223 (-109.3336, 75.979) -> (-106.7502, 75.979)
  line L224 (-106.7502, 75.979) -> (-106.7502, 76.3193)
  line L225 (-106.7502, 76.3193) -> (-106.332, 76.3193)
  line L226 (-106.332, 76.3193) -> (-106.332, 75.979)
  line L227 (-106.332, 75.979) -> (-106.2315, 75.979)
  spline S200 degree 2 poles (-106.2315, 75.979) (-105.6934, 75.979) (-105.1294, 75.4571) (-105.1294, 74.9708) knots 0 0 0 1 2 2 2
  spline S201 degree 2 poles (-105.1294, 74.9708) (-105.1294, 74.8315) (-105.1586, 74.5624) (-105.178, 74.4522) knots 0 0 0 1 2 2 2
  line L228 (-105.178, 74.4522) -> (-105.6416, 74.4522)
  line L229 (-109.3336, 69.6062) -> (-109.3336, 70.2966)
  line L230 (-109.3336, 70.2966) -> (-107.473, 71.7585)
  line L231 (-107.473, 71.7585) -> (-107.7356, 71.9919)
  line L232 (-107.7356, 71.9919) -> (-109.3336, 71.9919)
  line L233 (-109.3336, 71.9919) -> (-109.3336, 72.5235)
  line L234 (-109.3336, 72.5235) -> (-105.3336, 72.5235)
  line L235 (-105.3336, 72.5235) -> (-105.3336, 71.9919)
  line L236 (-105.3336, 71.9919) -> (-107.1716, 71.9919)
  line L237 (-107.1716, 71.9919) -> (-105.3336, 70.3517)
  line L238 (-105.3336, 70.3517) -> (-105.3336, 69.7034)
  line L239 (-105.3336, 69.7034) -> (-107.1197, 71.3598)
  line L240 (-107.1197, 71.3598) -> (-109.3336, 69.6062)
  line L241 (-109.3336, 68.812) -> (-109.3336, 69.3177)
  line L242 (-109.3336, 69.3177) -> (-106.332, 69.3177)
  line L243 (-106.332, 69.3177) -> (-106.332, 68.812)
  line L244 (-106.332, 68.812) -> (-109.3336, 68.812)
  line L245 (-105.8328, 68.7764) -> (-105.8328, 69.3501)
  line L246 (-105.8328, 69.3501) -> (-105.3077, 69.3501)
  line L247 (-105.3077, 69.3501) -> (-105.3077, 68.7764)
  line L248 (-105.3077, 68.7764) -> (-105.8328, 68.7764)
  spline S202 degree 2 poles (-109.392, 67.1621) (-109.392, 67.5738) (-108.922, 68.0373) (-108.4131, 68.0373) knots 0 0 0 1 2 2 2
  line L249 (-108.4131, 68.0373) -> (-106.7502, 68.0373)
  line L250 (-106.7502, 68.0373) -> (-106.7502, 68.3777)
  line L251 (-106.7502, 68.3777) -> (-106.332, 68.3777)
  line L252 (-106.332, 68.3777) -> (-106.332, 68.0373)
  line L253 (-106.332, 68.0373) -> (-105.4698, 68.0373)
  line L254 (-105.4698, 68.0373) -> (-105.4698, 67.5316)
  line L255 (-105.4698, 67.5316) -> (-106.332, 67.5316)
  line L256 (-106.332, 67.5316) -> (-106.332, 66.6013)
  line L257 (-106.332, 66.6013) -> (-106.7502, 66.6013)
  line L258 (-106.7502, 66.6013) -> (-106.7502, 67.5316)
  line L259 (-106.7502, 67.5316) -> (-108.1797, 67.5316)
  spline S203 degree 2 poles (-108.1797, 67.5316) (-108.4066, 67.5316) (-108.6562, 67.5154) (-108.7631, 67.4603) knots 0 0 0 1 2 2 2
  spline S204 degree 2 poles (-108.7631, 67.4603) (-108.8571, 67.4149) (-108.9511, 67.2107) (-108.9511, 67.0357) knots 0 0 0 1 2 2 2
  spline S205 degree 2 poles (-108.9511, 67.0357) (-108.9511, 66.9125) (-108.8766, 66.6824) (-108.8539, 66.6305) knots 0 0 0 1 2 2 2
  line L260 (-108.8539, 66.6305) -> (-108.8539, 66.6013)
  line L261 (-108.8539, 66.6013) -> (-109.3077, 66.6013)
  spline S206 degree 2 poles (-109.3077, 66.6013) (-109.3466, 66.7439) (-109.392, 67.0357) (-109.392, 67.1621) knots 0 0 0 1 2 2 2
  line L262 (-105.6367, 51.5559) -> (-110.1367, 53.1057)
  line L263 (-110.1367, 53.1057) -> (-110.1367, 53.7512)
  line L264 (-110.1367, 53.7512) -> (-105.6367, 55.301)
  line L265 (-105.6367, 55.301) -> (-105.6367, 54.6592)
  line L266 (-105.6367, 54.6592) -> (-109.3745, 53.412)
  line L267 (-109.3745, 53.412) -> (-105.6367, 52.1649)
  line L268 (-105.6367, 52.1649) -> (-105.6367, 51.5559)
  line L269 (-110.1367, 48.4781) -> (-110.1367, 51.2532)
  line L270 (-110.1367, 51.2532) -> (-109.4985, 51.2532)
  spline S207 degree 2 poles (-109.4985, 51.2532) (-109.2177, 50.9542) (-108.6963, 50.4218) (-108.4155, 50.1665) knots 0 0 0 1 2 2 2
  spline S208 degree 2 poles (-108.4155, 50.1665) (-107.8502, 49.6523) (-107.1719, 49.2767) (-106.8109, 49.2767) knots 0 0 0 1 2 2 2
  spline S209 degree 2 poles (-106.8109, 49.2767) (-106.6213, 49.2767) (-106.3369, 49.3934) (-106.2457, 49.4991) knots 0 0 0 1 2 2 2
  spline S210 degree 2 poles (-106.2457, 49.4991) (-106.1545, 49.6049) (-106.0634, 49.882) (-106.0634, 50.0498) knots 0 0 0 1 2 2 2
  spline S211 degree 2 poles (-106.0634, 50.0498) (-106.0634, 50.2103) (-106.1436, 50.5385) (-106.2056, 50.688) knots 0 0 0 1 2 2 2
  spline S212 degree 2 poles (-106.2056, 50.688) (-106.2566, 50.8156) (-106.4025, 51.0526) (-106.4535, 51.1256) knots 0 0 0 1 2 2 2
  line L271 (-106.4535, 51.1256) -> (-106.4535, 51.1584)
  line L272 (-106.4535, 51.1584) -> (-105.8117, 51.1584)
  spline S213 degree 2 poles (-105.8117, 51.1584) (-105.7206, 50.9724) (-105.5419, 50.3051) (-105.5419, 50.006) knots 0 0 0 1 2 2 2
  spline S214 degree 2 poles (-105.5419, 50.006) (-105.5419, 49.3752) (-106.2092, 48.6641) (-106.7781, 48.6641) knots 0 0 0 1 2 2 2
  spline S215 degree 2 poles (-106.7781, 48.6641) (-107.0443, 48.6641) (-107.4892, 48.788) (-107.6788, 48.8974) knots 0 0 0 1 2 2 2
  spline S216 degree 2 poles (-107.6788, 48.8974) (-107.8758, 49.0068) (-108.2623, 49.3241) (-108.4483, 49.4991) knots 0 0 0 1 2 2 2
  spline S217 degree 2 poles (-108.4483, 49.4991) (-108.7582, 49.7836) (-109.4219, 50.4801) (-109.6152, 50.688) knots 0 0 0 1 2 2 2
  line L273 (-109.6152, 50.688) -> (-109.6152, 48.4781)
  line L274 (-109.6152, 48.4781) -> (-110.1367, 48.4781)
  line L275 (-110.1367, 46.91) -> (-110.1367, 47.632)
  line L276 (-110.1367, 47.632) -> (-109.2761, 47.632)
  line L277 (-109.2761, 47.632) -> (-109.2761, 46.91)
  line L278 (-109.2761, 46.91) -> (-110.1367, 46.91)
  spline S218 degree 2 poles (-107.8867, 43.2013) (-109.0974, 43.2013) (-110.2315, 43.9051) (-110.2315, 44.6381) knots 0 0 0 1 2 2 2
  spline S219 degree 2 poles (-110.2315, 44.6381) (-110.2315, 45.382) (-109.0755, 46.0786) (-107.8903, 46.0786) knots 0 0 0 1 2 2 2
  spline S220 degree 2 poles (-107.8903, 46.0786) (-106.6723, 46.0786) (-105.5455, 45.3748) (-105.5455, 44.6381) knots 0 0 0 1 2 2 2
  spline S221 degree 2 poles (-105.5455, 44.6381) (-105.5455, 43.8979) (-106.7125, 43.2013) (-107.8867, 43.2013) knots 0 0 0 1 2 2 2
  spline S222 degree 2 poles (-109.2578, 43.9744) (-109.0354, 43.8869) (-108.3498, 43.814) (-107.8867, 43.814) knots 0 0 0 1 2 2 2
  spline S223 degree 2 poles (-107.8867, 43.814) (-107.4236, 43.814) (-106.7416, 43.8869) (-106.5119, 43.9781) knots 0 0 0 1 2 2 2
  spline S224 degree 2 poles (-106.5119, 43.9781) (-106.2822, 44.0692) (-106.0451, 44.3865) (-106.0451, 44.6381) knots 0 0 0 1 2 2 2
  spline S225 degree 2 poles (-106.0451, 44.6381) (-106.0451, 44.8897) (-106.2822, 45.2143) (-106.5192, 45.3091) knots 0 0 0 1 2 2 2
  spline S226 degree 2 poles (-106.5192, 45.3091) (-106.7489, 45.4003) (-107.4491, 45.4659) (-107.8903, 45.4659) knots 0 0 0 1 2 2 2
  spline S227 degree 2 poles (-107.8903, 45.4659) (-108.3644, 45.4659) (-108.9989, 45.4076) (-109.2469, 45.3128) knots 0 0 0 1 2 2 2
  spline S228 degree 2 poles (-109.2469, 45.3128) (-109.4803, 45.2252) (-109.7319, 44.9007) (-109.7319, 44.6381) knots 0 0 0 1 2 2 2
  spline S229 degree 2 poles (-109.7319, 44.6381) (-109.7319, 44.3902) (-109.4949, 44.0656) (-109.2578, 43.9744) knots 0 0 0 1 2 2 2
  spline S230 degree 2 poles (-97.3737, -47.9037) (-97.9215, -47.9037) (-98.8032, -47.4596) (-99.0495, -47.0869) knots 0 0 0 1 2 2 2
  spline S231 degree 2 poles (-99.0495, -47.0869) (-99.2408, -46.7822) (-99.3704, -46.1566) (-99.3704, -45.6703) knots 0 0 0 1 2 2 2
  line L279 (-99.3704, -45.6703) -> (-99.3704, -44.7498)
  line L280 (-99.3704, -44.7498) -> (-95.3704, -44.7498)